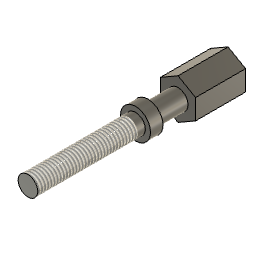
연습예제_4 (Autodesk Fusion 360 design; units mm, degrees)
Autodesk Fusion 360 part; units mm, degrees
sketch "Sketch3" plane through (0, 0, 0) normal (0, 1, 0) x (1, 0, 0)
  line L0 (7, 4.0415) -> (0, 8.0829)
  line L1 (0, 8.0829) -> (-7, 4.0415)
  line L2 (-7, 4.0415) -> (-7, -4.0415)
  line L3 (-7, -4.0415) -> (0, -8.0829)
  line L4 (0, -8.0829) -> (7, -4.0415)
  line L5 (7, -4.0415) -> (7, 4.0415)
  dimension "d5" = 14
  measures "d5" distance of L2 L5
extrude "Extrude2" add sketch "Sketch3" along normal blind 20
sketch "Sketch4" plane through (0, 0, 0) normal (0, -1, 0) x (1, 0, 0)
  circle A0 centre (0, 0) radius 4
  dimension "d8" = 8
  constraint coincident A0.centre origin
  measures "d8" diameter of A0
extrude "Extrude4" add sketch "Sketch4" along normal blind 12
sketch "Sketch5" plane through (0, -12, 0) normal (0, -1, 0) x (1, 0, 0)
  circle A0 centre (0, 0) radius 6
  dimension "d13" = 12
  constraint coincident A0.centre origin
  measures "d13" diameter of A0
extrude "Extrude5" add sketch "Sketch5" along normal blind 5
sketch "Sketch6" plane through (0, -17, 0) normal (0, -1, 0) x (1, 0, 0)
  circle A0 centre (0, 0) radius 4
  constraint coincident A0.centre origin
extrude "Extrude6" add sketch "Sketch6" along normal blind 43
thread "Thread2" "ISO Metric profile 8.0 M8x1.25 6g" major diameter 7.866 minor diameter 6.4455 pitch 1.25 angle 60 resizes the face on face at (3.995, -45.6667, -0.1994) from (0, -20, 0) to (0, -60, 0)
thread "Thread1" [suppressed]
extrude "Extrude3" [suppressed]
